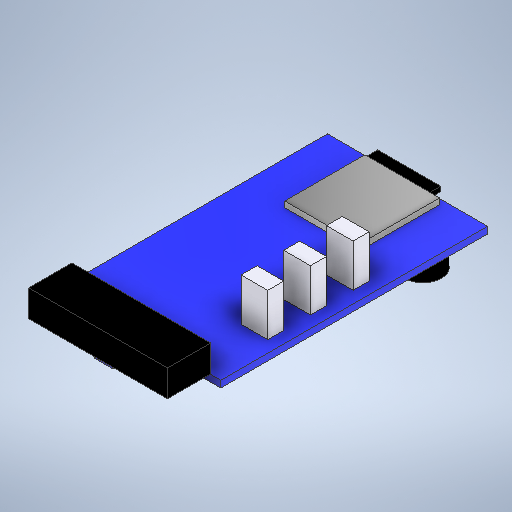
# Autodesk Inventor part: Sd card reader
Saved by Autodesk Inventor 2025.2 (Build 292293000, 293)
## iProperties
Created: 2025-04-04
Part Number: Sd card reader
Material: Generic
Document SubType Name: Modeling
Designer: joaki
Density: 1 g/cm^3
Appearance: Default
Author: joaki
Autodesk Inventor part; units mm, degrees
ref_plane "YZ Plane" through (0, 0, 0) normal (1, 0, 0) x (0, 1, 0)
ref_plane "XZ Plane" through (0, 0, 0) normal (0, 1, 0) x (-1, 0, 0)
ref_plane "XY Plane" through (0, 0, 0) normal (0, 0, 1) x (1, 0, 0)
sketch "Sketch1" plane through (0, 0, 0) normal (0, 1, 0) x (-1, 0, 0)
  line L0 (22.7568, 36.7979) -> (-7.2432, 36.7979)
  line L1 (-7.2432, 36.7979) -> (-7.2432, -13.2021)
  line L2 (-7.2432, -13.2021) -> (22.7568, -13.2021)
  line L3 (22.7568, -13.2021) -> (22.7568, 36.7979)
  line L4 (7.7568, 36.7979) -> (7.7568, 43.7979)
  line L5 (7.7568, 43.7979) -> (9.5068, 43.7979)
  line L6 (9.5068, 43.7979) -> (9.5068, 36.7979)
  line L7 (9.5068, 43.7979) -> (6.0068, 43.7979)
  line L8 (6.0068, 43.7979) -> (6.0068, 36.7979)
  point P0 (0, 0)
  dimension "d0" = 30
  dimension "d1" = 50
  dimension "d2" = 7
  dimension "d3" = 1.75
  dimension "d4" = 3.5
  constraints: 18 end point, 3 perpendicular, 3 point on line, 2 horizontal, 2 parallel, 1 midpoint, 1 vertical
  measures "d0" distance of L1.end L2.end
  measures "d1" distance of L2.end L0.start
  measures "d2" distance of L4.start L4.end
  measures "d3" distance of L4.end L5.end
  measures "d4" distance of L5.end L7.end
extrude "Extrusion1" add sketch "Sketch1" along normal blind 1.25
sketch "Sketch2" plane through (0, 1.25, 0) normal (0, 1, 0) x (1, 0, 0)
  line L0 (-20.7568, -36.6979) -> (5.2432, -36.6979)
  line L1 (5.2432, -36.6979) -> (5.2432, -44.7979)
  line L2 (5.2432, -44.7979) -> (-20.7568, -44.7979)
  line L3 (-20.7568, -44.7979) -> (-20.7568, -36.6979)
  line L4 (-9.5068, -43.7979) -> (-6.0068, -43.7979) projected
  line L5 (-6.0068, -43.7979) -> (-9.5068, -43.7979)
  line L6 (-22.7568, 13.2021) -> (-22.7568, -36.7979) projected
  line L7 (7.2432, -36.7979) -> (7.2432, 13.2021) projected
  point P0 (0, 0)
  point P1 (-7.7568, -43.7979)
  point P2 (5.2432, -40.7479)
  dimension "d7" = 1
  dimension "d8" = 8.1
  dimension "d9" = 2
  dimension "d10" = 2
  constraints: 10 end point, 2 horizontal, 2 midpoint, 2 parallel, 1 perpendicular
  measures "d7" distance from line of L2 point (-7.757, -43.798)
  measures "d8" distance between parallel lines of L0 L2
  measures "d9" distance between parallel lines of L6 L3
  measures "d10" distance from line of L7 point (5.243, -40.748)
extrude "Extrusion2" add sketch "Sketch2" along normal blind 5
sketch "Sketch3" plane through (0, 1.25, 0) normal (0, 1, 0) x (1, 0, 0)
  line L0 (0.0432, -9.7979) -> (5.0432, -9.7979)
  line L1 (5.0432, -9.7979) -> (5.0432, -6.7979)
  line L2 (5.0432, -6.7979) -> (0.0432, -6.7979)
  line L3 (0.0432, -6.7979) -> (0.0432, -9.7979)
  line L4 (0.0432, -17.7979) -> (5.0432, -17.7979)
  line L5 (5.0432, -17.7979) -> (5.0432, -14.7979)
  line L6 (5.0432, -14.7979) -> (0.0432, -14.7979)
  line L7 (0.0432, -14.7979) -> (0.0432, -17.7979)
  line L8 (0.0432, -25.7979) -> (5.0432, -25.7979)
  line L9 (5.0432, -25.7979) -> (5.0432, -22.7979)
  line L10 (5.0432, -22.7979) -> (0.0432, -22.7979)
  line L11 (0.0432, -22.7979) -> (0.0432, -25.7979)
  line L12 (7.2432, -36.7979) -> (7.2432, 13.2021) projected
  line L13 (7.2432, 13.2021) -> (-22.7568, 13.2021) projected
  point P0 (0, 0)
  point P1 (-0.1282, -6.8631)
  point P2 (-0.0024, -12.7771)
  point P3 (5.0432, -8.2979)
  point P4 (5.0432, -16.2979)
  point P5 (5.0432, -24.2979)
  point P6 (2.5432, -17.7979)
  point P7 (2.5432, -22.7979)
  dimension "d13" = 5
  dimension "d14" = 3
  dimension "d15" = 5
  dimension "d16" = 3
  dimension "d17" = 5
  dimension "d18" = 3
  dimension "d19" = 2.2
  dimension "d20" = 2.2
  dimension "d21" = 2.2
  dimension "d22" = 20
  dimension "d23" = 5
  dimension "d24" = 5
  constraints: 24 end point, 6 parallel, 5 midpoint, 3 horizontal, 3 perpendicular
  measures "d13" distance of L1.end L2.end
  measures "d14" distance of L0.end L1.end
  measures "d15" distance of L5.end L6.end
  measures "d16" distance of L4.end L5.end
  measures "d17" distance of L9.end L10.end
  measures "d18" distance of L8.end L9.end
  measures "d19" distance from line of L12 point (5.043, -8.298)
  measures "d20" distance from line of L12 point (5.043, -16.298)
  measures "d21" distance from line of L12 point (5.043, -24.298)
  measures "d22" distance between parallel lines of L13 L2
  measures "d23" distance between parallel lines of L6 L0
  measures "d24" distance of point (2.543, -17.798) point (2.543, -22.798)
extrude "Extrusion3" add sketch "Sketch3" along normal blind 8
sketch "Sketch4" plane through (0, 1.25, 0) normal (0, 1, 0) x (1, 0, 0)
  line L0 (-14.7568, -2.7979) -> (-0.7568, -2.7979)
  line L1 (-0.7568, -2.7979) -> (-0.7568, 12.2021)
  line L2 (-0.7568, 12.2021) -> (-14.7568, 12.2021)
  line L3 (-14.7568, 12.2021) -> (-14.7568, -2.7979)
  line L4 (-22.7568, 13.2021) -> (-22.7568, -36.7979) projected
  line L5 (7.2432, -36.7979) -> (7.2432, 13.2021) projected
  line L6 (7.2432, 13.2021) -> (-22.7568, 13.2021) projected
  point P0 (0, 0)
  dimension "d27" = 8
  dimension "d28" = 8
  dimension "d29" = 1
  dimension "d30" = 15
  constraints: 8 end point, 2 parallel, 1 horizontal, 1 perpendicular
  measures "d27" distance between parallel lines of L4 L3
  measures "d28" distance between parallel lines of L5 L1
  measures "d29" distance between parallel lines of L6 L2
  measures "d30" distance between parallel lines of L0 L2
extrude "Extrusion4" add sketch "Sketch4" along normal blind 1.1
sketch "Sketch5" plane through (-0.7568, 1.25, -12.2021) normal (0, 0, -1) x (-1, 0, 0)
  line L0 (2, 0.9) -> (13.8, 0.9)
  line L1 (13.8, 0.9) -> (13.8, 0.017)
  line L2 (13.8, 0.017) -> (2, 0.017)
  line L3 (2, 0.017) -> (2, 0.9)
  line L4 (0, 0) -> (0, 1.1) projected
  line L5 (14, 0) -> (14, 1.1) projected
  line L6 (0, 1.1) -> (14, 1.1) projected
  line L7 (-8, 0) -> (22, 0) projected
  point P0 (-0.7568, -1.25)
  point P1 (0, 0.55)
  point P2 (2, 0.4585)
  point P3 (14, 0.55)
  point P4 (13.8, 0.4585)
  dimension "d33" = 2
  dimension "d34" = 0.2
  dimension "d35" = 0.2
  dimension "d36" = 0.017
  constraints: 8 end point, 4 midpoint, 2 parallel, 1 horizontal, 1 perpendicular
  measures "d33" horizontal distance of point (0, 0.55) point (2, 0.458)
  measures "d34" horizontal distance of point (14, 0.55) point (13.8, 0.459)
  measures "d35" distance between parallel lines of L6 L0
  measures "d36" distance between parallel lines of L7 L2
extrude "Extrusion5" add sketch "Sketch5" along normal blind 2.2 contours L0 L1 L2 L3
sketch "Sketch6" plane through (0, 0, 0) normal (0, -1, 0) x (1, 0, 0)
  circle A0 centre (3.6432, -4.7021) radius 3.5
  circle A1 centre (-19.1568, -4.7021) radius 3.5
  line L0 (7.2432, -13.2021) -> (-22.7568, -13.2021) projected
  line L1 (-22.7568, -13.2021) -> (-22.7568, 36.7979) projected
  line L2 (7.2432, 36.7979) -> (7.2432, -13.2021) projected
  point P0 (0, 0)
  dimension "d39" = 7
  dimension "d40" = 7
  dimension "d41" = 8.5
  dimension "d42" = 8.5
  dimension "d43" = 3.6
  dimension "d44" = 3.6
  constraints: 2 centre point
  measures "d39" diameter of A0
  measures "d40" diameter of A1
  measures "d41" distance from line of L0 A0.centre
  measures "d42" distance from line of L0 A1.centre
  measures "d43" distance from line of L1 A1.centre
  measures "d44" distance from line of L2 A0.centre
extrude "Extrusion6" add sketch "Sketch6" along normal blind 3
body "Solid1"
